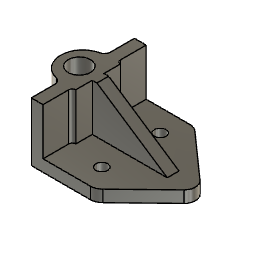
Homework2_A3_v2 (Autodesk Fusion 360 design; units mm, degrees)
Autodesk Fusion 360 part; units mm, degrees
note: some values were not read from the file. Set by a fixed rule: which sketch regions a step uses.
sketch "Sketch1" plane through (0, 0, 0) normal (0, 0, 1) x (1, 0, 0)
  line L0 (10, 88) -> (0, 88)
  line L1 (0, 0) -> (10, 0)
  line L2 (10, 0) -> (10, 22)
  line L3 (13, 25) -> (13, 25)
  line L4 (13, 25) -> (13, 39)
  line L5 (13, 39) -> (17, 39)
  line L6 (17, 39) -> (17, 49)
  line L7 (17, 49) -> (13, 49)
  line L8 (13, 49) -> (13, 63)
  line L9 (13, 63) -> (13, 63)
  line L10 (10, 66) -> (10, 88)
  arc A0 (10, 64) -> (11, 63) centre (11, 64) ccw
  line L11 (0, 0) -> (0, 20.5266)
  line L12 (0, 88) -> (0, 67.4734)
  arc A1 (-3.9583, 62.5831) -> (-3.9583, 25.4169) centre (0, 44) ccw
  arc A2 (0, 20.5266) -> (-3.9583, 25.4169) centre (-5, 20.5266) ccw
  arc A3 (-3.9583, 62.5831) -> (0, 67.4734) centre (-5, 67.4734) ccw
  arc A4 (10, 66) -> (13, 63) centre (13, 66) ccw
  arc A5 (13, 25) -> (10, 22) centre (13, 22) ccw
  dimension "d2" = 5
  dimension "d37" = 3
  dimension "d38" = 3
  constraint coincident L1.start L11.start
  constraint perpendicular L1 L2
  constraint perpendicular L4 L5
  constraint perpendicular L5 L6
  constraint perpendicular L4 L7
  constraint perpendicular L5 L8
  constraint perpendicular L0 L10
  constraint tangent L10 A0
  constraint perpendicular L1 L11
  constraint perpendicular L0 L12
  constraint tangent L11 A2
  constraint tangent A1 A2
  constraint tangent L12 A3
  constraint tangent A1 A3
  constraint equal A2 A3
  constraint coincident L10 A0.start
  constraint coincident L9 A0.end
  constraint tangent L10 A4
  constraint tangent L2 A5
  measures "d2" radius of A2
  measures "d37" radius of A4
  measures "d38" radius of A5
extrude "Extrude1" add sketch "Sketch1" along normal blind 50 makes body 1
hole "Hole1" at (-2.9996, 44.0006, 50) direction (0, 0, -1) diameter 19 depth 50 tip angle 118 bodies 1
sketch "Sketch2" plane through (0, 0, 0) normal (0, 1, 0) x (1, 0, 0)
  line L0 (17, -50) -> (17, -10)
  line L1 (17, -10) -> (77, -10)
  line L2 (77, -10) -> (17, -50)
  constraint vertical L0
  constraint perpendicular L0 L1
extrude "Extrude2" add sketch "Sketch2" along normal blind 10 separate body makes body 2
move_body "Move1" bodies 2 to x (1, 0, 0) y (0, 1, 0) z (0, 0, 1) at (0, 39, 0)
sketch "Sketch3" plane through (0, 0, 0) normal (0, 0, 1) x (1, 0, 0)
  line L0 (10, 88) -> (47.4072, 88)
  line L1 (50.3213, 0) -> (10, 0)
  line L2 (10, 0) -> (10, 88)
  line L3 (77, 20.475) -> (77, 20)
  line L4 (96, 44.0013) -> (96, 43.9987)
  line L5 (57.9798, 3.1039) -> (93.1141, 37.1806)
  arc A0 (50.3213, 0) -> (57.9798, 3.1039) centre (50.3213, 11) ccw
  arc A1 (93.1141, 37.1806) -> (92.1496, 51.6375) centre (86.5, 44) ccw
  line L6 (93.1141, 50.8194) -> (54.0436, 85.4806)
  arc A2 (54.0436, 85.4806) -> (47.4072, 88) centre (47.4072, 78) ccw
  dimension "d11" = 11
  dimension "d12" = 10
  constraint horizontal L0
  constraint horizontal L1
  constraint vertical L2
  constraint vertical L3
  constraint coincident L4.start A1
  constraint coincident L4.end A1
  constraint tangent L5 A1
  constraint tangent L1 A0
  constraint tangent L5 A0
  constraint coincident A1 L6.start
  constraint tangent L0 A2
  constraint tangent L6 A2
  measures "d11" radius of A0
  measures "d12" radius of A2
extrude "Extrude3" add sketch "Sketch3" along normal blind 10 contours L0 L1 L2 L4 L5 A0 A1 L6 A2 bodies 1 2
hole "Hole2" at (41.1971, 19.002, 10) direction (0, 0, -1) diameter 10 depth 10 tip angle 118 bodies 1
hole "Hole3" at (40.9034, 69.0011, 10) direction (0, 0, -1) diameter 10 depth 10 tip angle 118 bodies 1
move_body "Move2" bodies 1 to x (1, 0, 0) y (0, 1, 0) z (0, 0, 1) at (-180, 0, 0)
move_body "Move5" bodies 1 to x (1, 0, 0) y (0, 1, 0) z (0, 0, 1) at (0, -122, 0)
sketch "Sketch7" plane through (0, 0, 0) normal (0, 0, 1) x (1, 0, 0)
named bodies: "A3"
